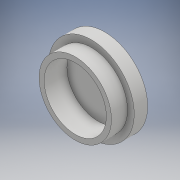
# Autodesk Inventor part: CapForPh
Saved by Autodesk Inventor 2019 (Build 230136000, 136)
## iProperties
Created: 2017-07-24
Part Number: CapForPh
Material: Generic
Document SubType Name: Modeling
Designer: steele
Density: 1 g/cm^3
Appearance: Default
Author: steele
Autodesk Inventor part; units mm, degrees
ref_plane "YZ Plane" through (0, 0, 0) normal (1, 0, 0) x (0, 1, 0)
ref_plane "XZ Plane" through (0, 0, 0) normal (0, 1, 0) x (-1, 0, 0)
ref_plane "XY Plane" through (0, 0, 0) normal (0, 0, 1) x (1, 0, 0)
sketch "Sketch2" plane through (0, 0, 0) normal (0, 0, 1) x (1, 0, 0)
  line L0 (0, 0) -> (0, 11) construction
  line L1 (0, 11) -> (-16, 11)
  line L2 (-16, 11) -> (-16, 6)
  line L3 (-16, 6) -> (-13.5, 6)
  line L4 (-13.5, 6) -> (-13.5, 0)
  line L5 (-13.5, 0) -> (-11.6, 0)
  line L6 (0, 0) -> (-13.5, 0) construction
  line L7 (-11.6, 0) -> (-11.6, 6)
  line L8 (0, 11) -> (0, 8.5)
  line L9 (-11.6, 8.5) -> (-11.6, 6)
  line L10 (-11.6, 8.5) -> (0, 8.5)
  dimension "d4" = 16
  dimension "d5" = 5
  dimension "d6" = 6
  dimension "d8" = 13.5
  dimension "d16" = 11.6
  constraints: 22 end point, 5 perpendicular, 3 vertical, 2 point on line, 1 collinear, 1 horizontal, 1 parallel
  measures "d4" distance of L0.end L1.end
  measures "d5" distance of L1.end L2.end
  measures "d6" distance of L3.end L4.end
  measures "d8" distance between parallel lines of L0 L4
  measures "d16" distance between parallel lines of L7 L0
revolve "Revolution1" add sketch "Sketch2" angle 360 about axis through (0, 0, 0) along (0, 1, 0)
sketch "Sketch4" plane through (0, 11, 0) normal (0, 1, 0) x (1, 0, 0)
  circle A0 centre (0, 0) radius 16 construction
  line L0 (-16, 0) -> (16, 0) construction
  spline S0 degree 2 poles (-8.5271, 1.2611) (-8.5271, 0.8656) (-8.8089, 0.1538) (-9.061, -0.0934) knots 0 0 0 1 2 2 2
  spline S1 degree 2 poles (-9.061, -0.0934) (-9.3774, -0.4048) (-10.2326, -0.7261) (-10.8851, -0.7261) knots 0 0 0 1 2 2 2
  line L1 (-10.8851, -0.7261) -> (-11.5722, -0.7261)
  line L2 (-11.5722, -0.7261) -> (-11.5722, -3)
  line L3 (-11.5722, -3) -> (-12.3829, -3)
  line L4 (-12.3829, -3) -> (-12.3829, 3.1)
  line L5 (-12.3829, 3.1) -> (-10.8505, 3.1)
  spline S2 degree 2 poles (-10.8505, 3.1) (-10.3067, 3.1) (-9.5455, 2.922) (-9.2538, 2.7194) knots 0 0 0 1 2 2 2
  spline S3 degree 2 poles (-9.2538, 2.7194) (-8.9127, 2.487) (-8.5271, 1.7703) (-8.5271, 1.2611) knots 0 0 0 1 2 2 2
  spline S4 degree 2 poles (-9.3724, 1.2364) (-9.3724, 1.5528) (-9.59, 2.0174) (-9.8124, 2.1657) knots 0 0 0 1 2 2 2
  spline S5 degree 2 poles (-9.8124, 2.1657) (-10.0052, 2.2942) (-10.5193, 2.3981) (-10.8999, 2.3981) knots 0 0 0 1 2 2 2
  line L6 (-10.8999, 2.3981) -> (-11.5722, 2.3981)
  line L7 (-11.5722, 2.3981) -> (-11.5722, -0.034)
  line L8 (-11.5722, -0.034) -> (-11.0186, -0.034)
  spline S6 degree 2 poles (-11.0186, -0.034) (-10.5242, -0.034) (-9.9162, 0.1241) (-9.7185, 0.3318) knots 0 0 0 1 2 2 2
  spline S7 degree 2 poles (-9.7185, 0.3318) (-9.5356, 0.5147) (-9.3724, 0.9447) (-9.3724, 1.2364) knots 0 0 0 1 2 2 2
  line L9 (-4.2216, -3) -> (-4.9927, -3)
  line L10 (-4.9927, -3) -> (-4.9927, -0.39)
  spline S8 degree 2 poles (-4.9927, -0.39) (-4.9927, -0.0736) (-5.052, 0.4702) (-5.141, 0.6333) knots 0 0 0 1 2 2 2
  spline S9 degree 2 poles (-5.141, 0.6333) (-5.2349, 0.8063) (-5.5711, 0.9744) (-5.8578, 0.9744) knots 0 0 0 1 2 2 2
  spline S10 degree 2 poles (-5.8578, 0.9744) (-6.1445, 0.9744) (-6.7525, 0.6679) (-7.0442, 0.4207) knots 0 0 0 1 2 2 2
  line L11 (-7.0442, 0.4207) -> (-7.0442, -3)
  line L12 (-7.0442, -3) -> (-7.8153, -3)
  line L13 (-7.8153, -3) -> (-7.8153, 3.3719)
  line L14 (-7.8153, 3.3719) -> (-7.0442, 3.3719)
  line L15 (-7.0442, 3.3719) -> (-7.0442, 1.0683)
  spline S11 degree 2 poles (-7.0442, 1.0683) (-6.6981, 1.3797) (-6.0308, 1.706) (-5.6551, 1.706) knots 0 0 0 1 2 2 2
  spline S12 degree 2 poles (-5.6551, 1.706) (-4.9828, 1.706) (-4.2216, 0.8162) (-4.2216, -0.0291) knots 0 0 0 1 2 2 2
  line L16 (-4.2216, -0.0291) -> (-4.2216, -3)
  spline S13 degree 2 poles (1.9229, -3.1088) (1.3297, -3.1088) (0.3263, -2.7083) (-0.0395, -2.3079) knots 0 0 0 1 2 2 2
  spline S14 degree 2 poles (-0.0395, -2.3079) (-0.4053, -1.9125) (-0.8058, -0.7261) (-0.8058, 0.0451) knots 0 0 0 1 2 2 2
  spline S15 degree 2 poles (-0.8058, 0.0451) (-0.8058, 0.8113) (-0.4152, 1.9482) (-0.0445, 2.3684) knots 0 0 0 1 2 2 2
  spline S16 degree 2 poles (-0.0445, 2.3684) (0.3213, 2.7787) (1.3199, 3.2088) (1.9378, 3.2088) knots 0 0 0 1 2 2 2
  spline S17 degree 2 poles (1.9378, 3.2088) (2.2442, 3.2088) (2.7831, 3.1198) (3.0105, 3.0506) knots 0 0 0 1 2 2 2
  spline S18 degree 2 poles (3.0105, 3.0506) (3.2082, 2.9863) (3.6185, 2.8034) (3.8212, 2.6947) knots 0 0 0 1 2 2 2
  line L17 (3.8212, 2.6947) -> (3.8212, 1.7159)
  line L18 (3.8212, 1.7159) -> (3.7569, 1.7159)
  spline S19 degree 2 poles (3.7569, 1.7159) (3.6481, 1.8147) (3.312, 2.0916) (3.0698, 2.225) knots 0 0 0 1 2 2 2
  spline S20 degree 2 poles (3.0698, 2.225) (2.8374, 2.3536) (2.2887, 2.5167) (1.9328, 2.5167) knots 0 0 0 1 2 2 2
  spline S21 degree 2 poles (1.9328, 2.5167) (1.5423, 2.5167) (0.8453, 2.1954) (0.5833, 1.8889) knots 0 0 0 1 2 2 2
  spline S22 degree 2 poles (0.5833, 1.8889) (0.3263, 1.5775) (0.0395, 0.6333) (0.0395, 0.0451) knots 0 0 0 1 2 2 2
  spline S23 degree 2 poles (0.0395, 0.0451) (0.0395, -0.5827) (0.3411, -1.4874) (0.6031, -1.7988) knots 0 0 0 1 2 2 2
  spline S24 degree 2 poles (0.6031, -1.7988) (0.8601, -2.1003) (1.5472, -2.4068) (1.9328, -2.4068) knots 0 0 0 1 2 2 2
  spline S25 degree 2 poles (1.9328, -2.4068) (2.2838, -2.4068) (2.8819, -2.2338) (3.1143, -2.1053) knots 0 0 0 1 2 2 2
  spline S26 degree 2 poles (3.1143, -2.1053) (3.3367, -1.9767) (3.6679, -1.7098) (3.7618, -1.6159) knots 0 0 0 1 2 2 2
  line L19 (3.7618, -1.6159) -> (3.8212, -1.6159)
  line L20 (3.8212, -1.6159) -> (3.8212, -2.5848)
  spline S27 degree 2 poles (3.8212, -2.5848) (3.6185, -2.6787) (3.2626, -2.8517) (3.0105, -2.9308) knots 0 0 0 1 2 2 2
  spline S28 degree 2 poles (3.0105, -2.9308) (2.7435, -3.0198) (2.2887, -3.1088) (1.9229, -3.1088) knots 0 0 0 1 2 2 2
  spline S29 degree 2 poles (7.0689, -2.5156) (6.975, -2.5848) (6.6586, -2.8319) (6.5103, -2.9061) knots 0 0 0 1 2 2 2
  spline S30 degree 2 poles (6.5103, -2.9061) (6.3076, -3.0148) (5.927, -3.1285) (5.581, -3.1285) knots 0 0 0 1 2 2 2
  spline S31 degree 2 poles (5.581, -3.1285) (5.2992, -3.1285) (4.79, -2.916) (4.5972, -2.7232) knots 0 0 0 1 2 2 2
  spline S32 degree 2 poles (4.5972, -2.7232) (4.4143, -2.5353) (4.1919, -1.9817) (4.1919, -1.6752) knots 0 0 0 1 2 2 2
  spline S33 degree 2 poles (4.1919, -1.6752) (4.1919, -1.2006) (4.5923, -0.5284) (5.0273, -0.3356) knots 0 0 0 1 2 2 2
  spline S34 degree 2 poles (5.0273, -0.3356) (5.4129, -0.1576) (6.4609, -0.0241) (7.0689, 0.0105) knots 0 0 0 1 2 2 2
  line L21 (7.0689, 0.0105) -> (7.0689, 0.1588)
  spline S35 degree 2 poles (7.0689, 0.1588) (7.0689, 0.4257) (6.9058, 0.7569) (6.7575, 0.8508) knots 0 0 0 1 2 2 2
  spline S36 degree 2 poles (6.7575, 0.8508) (6.6092, 0.9447) (6.184, 1.0041) (5.9566, 1.0041) knots 0 0 0 1 2 2 2
  spline S37 degree 2 poles (5.9566, 1.0041) (5.6897, 1.0041) (4.968, 0.8459) (4.6071, 0.6926) knots 0 0 0 1 2 2 2
  line L22 (4.6071, 0.6926) -> (4.5626, 0.6926)
  line L23 (4.5626, 0.6926) -> (4.5626, 1.4786)
  spline S38 degree 2 poles (4.5626, 1.4786) (4.7752, 1.5379) (5.5711, 1.6862) (5.9616, 1.6862) knots 0 0 0 1 2 2 2
  spline S39 degree 2 poles (5.9616, 1.6862) (6.4361, 1.6862) (7.0837, 1.5379) (7.3408, 1.3451) knots 0 0 0 1 2 2 2
  spline S40 degree 2 poles (7.3408, 1.3451) (7.5929, 1.1573) (7.84, 0.5592) (7.84, 0.1291) knots 0 0 0 1 2 2 2
  line L24 (7.84, 0.1291) -> (7.84, -3)
  line L25 (7.84, -3) -> (7.0689, -3)
  line L26 (7.0689, -3) -> (7.0689, -2.5156)
  line L27 (7.0689, -1.8729) -> (7.0689, -0.6025)
  spline S41 degree 2 poles (7.0689, -0.6025) (6.7921, -0.6272) (5.9566, -0.7113) (5.6947, -0.7904) knots 0 0 0 1 2 2 2
  spline S42 degree 2 poles (5.6947, -0.7904) (5.3882, -0.8843) (4.9878, -1.2748) (4.9878, -1.6208) knots 0 0 0 1 2 2 2
  spline S43 degree 2 poles (4.9878, -1.6208) (4.9878, -2.0163) (5.4327, -2.4167) (5.8578, -2.4167) knots 0 0 0 1 2 2 2
  spline S44 degree 2 poles (5.8578, -2.4167) (6.2186, -2.4167) (6.8118, -2.1053) (7.0689, -1.8729) knots 0 0 0 1 2 2 2
  spline S45 degree 2 poles (12.7586, -0.5877) (12.7586, -1.7345) (11.6661, -3.089) (10.8307, -3.089) knots 0 0 0 1 2 2 2
  spline S46 degree 2 poles (10.8307, -3.089) (10.4896, -3.089) (9.9656, -2.9308) (9.6938, -2.7677) knots 0 0 0 1 2 2 2
  line L28 (9.6938, -2.7677) -> (9.6938, -4.6857)
  line L29 (9.6938, -4.6857) -> (8.9226, -4.6857)
  line L30 (8.9226, -4.6857) -> (8.9226, 1.5775)
  line L31 (8.9226, 1.5775) -> (9.6938, 1.5775)
  line L32 (9.6938, 1.5775) -> (9.6938, 1.098)
  spline S47 degree 2 poles (9.6938, 1.098) (9.9805, 1.36) (10.6824, 1.706) (11.0927, 1.706) knots 0 0 0 1 2 2 2
  spline S48 degree 2 poles (11.0927, 1.706) (11.8787, 1.706) (12.7586, 0.4603) (12.7586, -0.5877) knots 0 0 0 1 2 2 2
  spline S49 degree 2 poles (11.9627, -0.6767) (11.9627, 0.1093) (11.4635, 0.9744) (10.9049, 0.9744) knots 0 0 0 1 2 2 2
  spline S50 degree 2 poles (10.9049, 0.9744) (10.5786, 0.9744) (9.9656, 0.6827) (9.6938, 0.4553) knots 0 0 0 1 2 2 2
  line L33 (9.6938, 0.4553) -> (9.6938, -2.1448)
  spline S51 degree 2 poles (9.6938, -2.1448) (9.9953, -2.2882) (10.4254, -2.3969) (10.7022, -2.3969) knots 0 0 0 1 2 2 2
  spline S52 degree 2 poles (10.7022, -2.3969) (11.3003, -2.3969) (11.9627, -1.517) (11.9627, -0.6767) knots 0 0 0 1 2 2 2
  point P0 (0, 0)
  constraints: 2 end point, 2 horizontal, 2 point on circle
extrude "Extrusion2" cut sketch "Sketch4" against normal blind 2
body "Solid1"
